mounter v234 (Autodesk Fusion 360 design; units mm, degrees)
Autodesk Fusion 360 part; units mm, degrees
note: some values were not read from the file. Set by a fixed rule: which sketch regions a step uses.
sketch "スケッチ1" plane through (0, 0, 0) normal (0, 0, 1) x (1, 0, 0)
  line L0 (0, 0) -> (18.0857, 0)
  line L1 (18.0857, 0) -> (18.0857, 13.2439)
  line L2 (18.0857, 13.2439) -> (0, 13.2439)
  line L3 (0, 13.2439) -> (0, 0)
  line L4 (0, 0) -> (-13.9996, 0)
  line L5 (-13.9996, 0) -> (-13.9996, 13.2439)
  line L6 (-13.9996, 13.2439) -> (0, 13.2439)
  line L7 (0, 13.2439) -> (0, 0)
  circle A0 centre (-6.9857, 4.9) radius 2
  circle A1 centre (6.9857, 4.9) radius 2
  circle A2 centre (0, 9) radius 2
  circle A3 centre (14.1857, 2.8) radius 3
  circle A4 centre (-6.9857, 4.9) radius 2.5
  circle A5 centre (6.9857, 4.9) radius 2.5
  circle A6 centre (0, 9) radius 2.3
  circle A7 centre (0, 9) radius 1.7
  line L8 (-7, 1.5) -> (-7, 0)
  line L9 (7, 1.5) -> (7, 0)
  circle A8 centre (-6.9857, 4.9) radius 3.4
  circle A9 centre (0, 9) radius 2.9
  line L10 (-6.9857, 4.9) -> (0, 9)
  line L11 (0, 9) -> (6.9857, 4.9)
  line L12 (6.9857, 4.9) -> (14.1857, 2.8)
  circle A10 centre (6.9857, 4.9) radius 3.4
  circle A11 centre (14.1857, 2.8) radius 3.9
  line L13 (-4.6, 2.4775) -> (-4.6, 0)
  line L14 (4.6, 2.4775) -> (4.6, 0)
  line L15 (-9.4, 2.506) -> (-9.4, 0)
  line L16 (9.4, 2.506) -> (9.4, 0)
  line L17 (-3.6347, 5.4753) -> (-1.6695, 6.6287)
  line L18 (1.6695, 6.6287) -> (3.6347, 5.4753)
  line L19 (-4.8495, 7.5452) -> (-2.8843, 8.6986)
  line L20 (2.8843, 8.6986) -> (4.8495, 7.5452)
  line L21 (10.2588, 5.8204) -> (11.3683, 5.4967)
  line L22 (9.2508, 2.3644) -> (10.3603, 2.0407)
  line L23 (0, 0) -> (18.0857, 0)
  line L24 (18.0857, 0) -> (18.0857, -2.0683)
  line L25 (18.0857, -2.0683) -> (0, -2.0683)
  line L26 (-13.9996, 0) -> (0, 0)
  line L27 (0, -2.0683) -> (-13.9996, -2.0683)
  line L28 (-13.9996, -2.0683) -> (-13.9996, 0)
  line L29 (-12.3, 6.4) -> (-12.3, 10)
  line L30 (-12.3, 10) -> (-8.7, 10)
  line L31 (-8.7, 10) -> (-8.7, 7.8362)
  line L32 (-12.3, 6.4) -> (-10.0369, 6.4)
  line L33 (-5.5, 1.65) -> (-8.5, 1.65)
  line L34 (-8.5, 1.65) -> (-8.5, 0.4)
  line L35 (-8.5, 0.4) -> (-5.5, 0.4)
  line L36 (-5.5, 0.4) -> (-5.5, 1.65)
  line L37 (-5.5, 1.65) -> (-8.5, 0.4) construction
  line L38 (-8.5, 1.65) -> (-5.5, 0.4) construction
  line L39 (8.5, 1.65) -> (5.5, 1.65)
  line L40 (5.5, 1.65) -> (5.5, 0.4)
  line L41 (5.5, 0.4) -> (8.5, 0.4)
  line L42 (8.5, 0.4) -> (8.5, 1.65)
  line L43 (8.5, 1.65) -> (5.5, 0.4) construction
  line L44 (5.5, 1.65) -> (8.5, 0.4) construction
  arc A12 (-12.3, 9.4) -> (-9.3, 6.4) centre (-9.3, 9.4) ccw
  point P0 (-7, 1.5)
  point P1 (7, 1.5)
  point P2 (-10.5, 10)
  point P3 (-7, 1.025)
  point P4 (7, 1.025)
  dimension "d4" = 4
  dimension "d5" = 4.9
  dimension "d6" = 8.1
  dimension "d7" = 4
  dimension "d10" = 6
  dimension "d16" = 2.8
  dimension "d18" = 9
  dimension "d19" = 5
  dimension "d21" = 7.5
  dimension "d26" = 4.6
  dimension "d34" = 3.4
  dimension "d41" = 7
  dimension "d45" = 5.8
  dimension "d51" = 1.2
  dimension "d52" = 4.8
  dimension "d54" = 1.8
  dimension "d57" = 6.8
  dimension "d76" = 7.8
  dimension "d86" = 10.5
  dimension "d87" = 3.6
  dimension "d88" = 10
  dimension "d92" = 3
  dimension "d93" = 0.4
  dimension "d94" = 1.25
  dimension "d96" = 3.6
  dimension "d97" = 3
  measures "d4" diameter of A0
  measures "d5" distance of L4 A0.centre
  measures "d6" distance of A0.centre A2.centre
  measures "d7" diameter of A2
  measures "d10" diameter of A3
  measures "d16" distance of L4 A3.centre
  measures "d18" distance of L0 A2.centre
  measures "d19" diameter of A4
  measures "d21" distance of A1.centre A3.centre
  measures "d26" diameter of A6
  measures "d34" diameter of A7
  measures "d41" distance of L7 P0
  measures "d45" diameter of A9
  measures "d51" distance of L10 L17
  measures "d52" distance of L13 L15
  measures "d54" distance of L12 L22
  measures "d57" diameter of A8
  measures "d76" diameter of A11
  measures "d86" distance of L3 P2
  measures "d87" distance of L29.end L30.end
  measures "d88" distance of L4.end L29.end
  measures "d92" distance of L34.end L35.end
  measures "d93" distance of L4 L35
  measures "d94" distance of L33.end L34.end
  measures "d96" distance of L29.start L29.end
  measures "d97" distance of L29 A12.centre
extrude "押し出し1" add sketch "スケッチ1" along normal blind 3 contours L0 L9 A10 L14 L23 L39 L40 L41 | L3 L7 A6 A9 L10 | L3 L7 A6 A9 L11 | L4 L8 A8 L13 L26 L33 L35 L36 | L0 L9 A10 L16 L22 L23 L39 L41 L42 | A5 L11 L12 A10 L39 | A8 A9 L10 L17 | A9 L11 A10 L18 | L4 L8 A8 L15 L26 L33 L34 L35 | A8 L33 | L3 L7 A6 A9 L10 | L3 L7 A6 A9 L11 | A8 A9 L10 L19 | A9 L11 A10 L20 | L0 A3 L12 A11 L23 | L0 A3 A11 L23 | A10 L16 L22 | L12 A10 A11 L16 L22 | A5 L11 L12 A10 | L0 A3 L12 A11 L23 | L12 A10 A11 L21 | A8 L29 L30 L31 A12 picked at (-7.0288, 1.9011)
extrude "押し出し2" add sketch "スケッチ1" along normal blind 0.5 contours A1 A5 L11 L12 | A1 A5 L11 L12 | A4
extrude "押し出し5" add sketch "スケッチ1" against normal blind 2.3 from surface at 3 contours L3 L7 A2 A6 L10 | L3 L7 A2 A6 L11 | L3 L7 A2 A6 L10 | L3 L7 A2 A6 L11
sketch "スケッチ2" plane through (0, 0, 0) normal (0, -1, 0) x (1, 0, 0)
  line L0 (-7, 0) -> (-7, 3)
  line L1 (7, 0) -> (7, 3)
  circle A0 centre (-7, 1.5) radius 0.8
  circle A1 centre (7, 1.5) radius 0.8
  line L2 (9.4, 0) -> (9.4, 3)
  line L3 (4.6, 3) -> (4.6, 0)
  line L4 (-4.6, 3) -> (-9.4, 3)
  line L5 (4.6, 0) -> (9.4, 0)
  line L6 (-4.6, 0) -> (-4.6, 3)
  line L7 (-9.4, 3) -> (-9.4, 0)
  line L8 (9.4, 3) -> (4.6, 3)
  line L9 (-9.4, 0) -> (-4.6, 0)
  point P0 (7, 0)
  dimension "d42" = 1.6
  measures "d42" diameter of A0
extrude "押し出し7" cut sketch "スケッチ2" against normal blind 3 contours L0 A0 | L0 A0 | L1 A1 | L1 A1
extrude "押し出し8" add sketch "スケッチ1" against normal blind 0.3 from surface at 1 contours L3 L7 A2 A7 L10 | L3 L7 A2 A7 L11 | L3 L7 A2 A7 L10 | L3 L7 A2 A7 L11
sketch "スケッチ6" plane through (0, 10, 0) normal (0, 1, 0) x (-1, 0, 0)
  line L0 (8.7, 0) -> (12.3, 0)
  line L1 (12.3, 0) -> (12.3, 3)
  line L2 (12.3, 3) -> (8.7, 3)
  line L3 (8.7, 3) -> (8.7, 0)
  line L4 (10.5, 3) -> (10.5, 0)
  circle A0 centre (10.5, 1.5) radius 0.75
  dimension "d89" = 1.5
  measures "d89" diameter of A0
extrude "押し出し12" cut sketch "スケッチ6" against normal blind 2.6 contours L4 A0 | L4 A0
equation "d5 = 6.5 mm - 0.6 mm - 1.0 mm"
equation "d6 = 6 mm + 2.0 mm + 0.1 mm"
equation "d16 = ( 7.8 / 2 ) * 1 mm - 0.6 mm - 0.5 mm"
equation "d21 = 6 mm + 1.4 mm + 0.1 mm"
